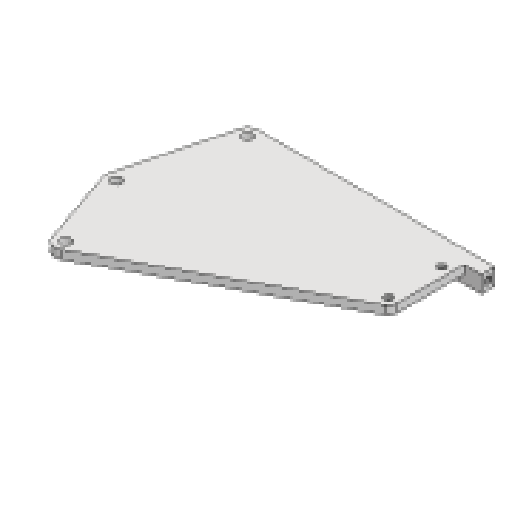
# Autodesk Inventor part: intakeSlidesWheelHolder
Saved by Autodesk Inventor 2023 (Build 270158000, 158)
## iProperties
Created: 2022-11-03
Part Number: intakeSlidesWheelHolder
Material: Generic
Document SubType Name: Modeling
Designer: deli
Density: 1 g/cm^3
Appearance: Default
Author: deli
Autodesk Inventor part; units mm, degrees
ref_plane "YZ Plane" through (0, 0, 0) normal (1, 0, 0) x (0, 1, 0)
ref_plane "XZ Plane" through (0, 0, 0) normal (0, 1, 0) x (-1, 0, 0)
ref_plane "XY Plane" through (0, 0, 0) normal (0, 0, 1) x (1, 0, 0)
sketch "Sketch1" plane through (0, 0, 0) normal (0, 1, 0) x (-1, 0, 0)
  circle A0 centre (23.0548, 41.1652) radius 1.5
  circle A1 centre (23.0548, 21.1652) radius 1.5
  arc A2 (26.5548, 41.1652) -> (19.5548, 41.1652) centre (23.0548, 41.1652) ccw
  line L0 (26.5548, 41.1652) -> (26.5548, 11.1652)
  line L1 (101.8798, 11.1652) -> (13.0548, 11.1652)
  line L2 (19.5548, 16.1652) -> (19.5548, 41.1652)
  line L3 (13.0548, 11.1652) -> (13.0548, 16.1652)
  line L4 (13.0548, 16.1652) -> (19.5548, 16.1652)
  circle A3 centre (112.0548, 54.1652) radius 2
  circle A4 centre (112.0548, 54.1652) radius 25 construction
  circle A5 centre (101.8798, 15.1652) radius 2
  circle A6 centre (101.8798, 83.4478) radius 2
  arc A7 (101.8798, 11.1652) -> (105.7503, 14.1554) centre (101.8798, 15.1652) ccw
  arc A8 (115.9253, 53.1554) -> (115.8332, 55.4781) centre (112.0548, 54.1652) ccw
  arc A9 (105.6582, 84.7607) -> (99.9694, 86.9621) centre (101.8798, 83.4478) ccw
  line L5 (105.7503, 14.1554) -> (115.9253, 53.1554)
  line L6 (115.8332, 55.4781) -> (105.6582, 84.7607)
  line L7 (21.3832, 44.2402) -> (99.9694, 86.9621)
  point P0 (0, 0)
  dimension "d0" = 3
  dimension "d1" = 2
  dimension "d2" = 20
  dimension "d3" = 10
  dimension "d20" = 10
  dimension "d28" = 4
  dimension "d29" = 85.5
  dimension "d30" = 3.5
  dimension "d32" = 5
  dimension "d33" = 50
  dimension "d34" = 4
  dimension "d35" = 75.325
  dimension "d36" = 75.325
  dimension "d38" = 4
  dimension "d39" = 8
  dimension "d40" = 39
  constraints: 16 end point, 10 centre point, 9 point on circle, 9 tangent, 5 coincident, 4 equal radius, 2 horizontal, 1 parallel, 1 perpendicular, 1 point on line, 1 vertical
  measures "d0" diameter of A0
  measures "d1" radial gap between concentric circles of A2 A0
  measures "d2" distance of A0.centre A1.centre
  measures "d3" distance from line of L1 A1.centre
  measures "d20" distance from line of A1.centre L3
  measures "d28" diameter of A3
  measures "d29" distance from line of L0 A3.centre
  measures "d30" distance from line of A1.centre L0
  measures "d32" distance of L1.end L3.end
  measures "d33" diameter of A4
  measures "d34" diameter of A5
  measures "d35" distance from line of L0 A5.centre
  measures "d36" distance from line of A6.centre L0
  measures "d39" diameter of A7
  measures "d40" vertical distance of A3.centre A5.centre
extrude "Extrusion1" add sketch "Sketch1" along normal blind 3.175
sketch "Sketch2" plane through (0, 3.175, 0) normal (0, 1, 0) x (1, 0, 0)
  line L0 (-26.6331, -11.1658) -> (-13.0548, -11.1658)
  line L1 (-13.0548, -11.1658) -> (-13.0548, -16.1652)
  line L2 (-13.0548, -16.1652) -> (-26.6331, -16.1652)
  line L3 (-26.6331, -16.1652) -> (-26.6331, -11.1658)
  point P0 (0, 0)
  constraints: 8 end point, 2 coincident, 2 parallel, 1 horizontal, 1 perpendicular
extrude "Extrusion2" add sketch "Sketch2" against normal blind 6.35
thread "Thread1" size "M3x0.5" class "6H" standard "ANSI Metric M Profile" full length
thread "Thread3" size "M3x0.5" class "6H" standard "ANSI Metric M Profile" full length
sketch "Sketch4" plane through (-13.0548, 0, 16.1652) normal (1, 0, 0) x (0, 0, -1)
  line L0 (-0.2072, 0) -> (-25.2049, 0) projected
  circle A0 centre (2.3958, 0) radius 1.5
  line L1 (0, 0) -> (0, -3.175) construction
  line L2 (4.7916, 3.175) -> (-25.2049, 3.175) construction
  line L3 (0, -3.175) -> (4.7916, 3.175) construction
  point P0 (16.1652, 0)
  dimension "d26" = 3
  constraints: 2 end point, 1 centre point, 1 coincident, 1 midpoint, 1 other
  measures "d26" diameter of A0
extrude "Extrusion4" cut sketch "Sketch4" against normal blind 8
thread "Thread4" size "M3x0.5" class "6H" standard "ANSI Metric M Profile" full length
equation "\"d36\" = d35"
body "Solid1"
